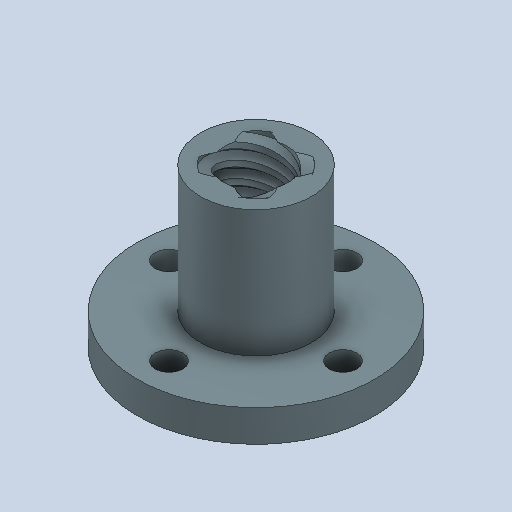
# Autodesk Inventor part: Nut
Saved by Autodesk Inventor 2024 (Build 280153000, 153)
## iProperties
Created: 2022-08-25
Part Number: Nut
Material: Lead
Document SubType Name: Modeling
Designer: Andrew
Density: 11.34 g/cm^3
Appearance: Lead
Author: Andrew
Autodesk Inventor part; units mm, degrees
ref_plane "YZ Plane" through (0, 0, 0) normal (1, 0, 0) x (0, 1, 0)
ref_plane "XZ Plane" through (0, 0, 0) normal (0, 1, 0) x (-1, 0, 0)
ref_plane "XY Plane" through (0, 0, 0) normal (0, 0, 1) x (1, 0, 0)
sketch "Sketch1" plane through (0, 0, 0) normal (0, 1, 0) x (-1, 0, 0)
  circle A0 centre (0, 0) radius 15
  circle A1 centre (0, 0) radius 11 construction
  circle A2 centre (0, 0) radius 7
  circle A3 centre (0, 0) radius 4
  circle A4 centre (11, 0) radius 1.75
  circle A5 centre (0, -11) radius 1.75
  circle A6 centre (-11, 0) radius 1.75
  circle A7 centre (0, 11) radius 1.75
  dimension "d1" = 22
  dimension "d0" = 30
  dimension "d2" = 14
  dimension "d3" = 8
  dimension "d4" = 3.5
  dimension "d7" = 360
  constraints: 7 centre point, 6 coincident, 1 horizontal alignment, 13 other
  measures "d0" diameter of A0
  measures "d2" diameter of A2
  measures "d3" diameter of A3
  measures "d4" diameter of A4
extrude "Extrusion1" add sketch "Sketch1" along normal blind 20 contours A2
extrude "Extrusion2" add sketch "Sketch1" along normal blind 4 contours A0
sketch "Sketch2" plane through (0, 0, 0) normal (1, 0, 0) x (0, 1, 0)
  line L0 (20, -2.634) -> (22, -2.634) construction
  line L1 (22, -2.634) -> (22, -6.366) construction
  line L2 (22, -6.366) -> (20, -6.366) construction
  line L3 (20, -6.366) -> (20, -2.634) construction
  line L4 (20, -4.5) -> (22, -4.5) construction
  line L5 (20, -4) -> (22, -4) construction
  line L6 (20, -3.75) -> (22, -3.75) construction
  line L7 (20, -5) -> (22, -5) construction
  line L8 (20, -5.25) -> (22, -5.25) construction
  line L9 (20, -2.634) -> (21, -6.366) construction
  line L10 (22, -2.634) -> (21, -6.366) construction
  line L11 (20.366, -4) -> (21.634, -4)
  line L12 (21.299, -5.25) -> (20.701, -5.25)
  line L13 (21.634, -4) -> (21.299, -5.25)
  line L14 (20.366, -4) -> (20.701, -5.25)
  line L15 (0, 0) -> (20, 0)
  line L16 (20, -7) -> (20, 7) projected
  dimension "d13" = 2
  dimension "d14" = 3.7321
  dimension "d15" = 0.5
  dimension "d16" = 0.75
  dimension "d17" = 9
  constraints: 32 end point, 12 point on line, 5 midpoint, 4 symmetric about line, 3 collinear, 3 perpendicular, 2 parallel, 1 horizontal
  measures "d13" distance of L2.start L3.start
  measures "d14" distance of L1.start L2.start
  measures "d15" distance between parallel lines of L5 L4
  measures "d16" distance between parallel lines of L6 L4
  measures "d17" diameter of L4 L15
coil "Coil1" sketch "Sketch2" operation cut axis through (0, 0, 0) along (0, -1, 0) pitch 8 turns 2.75 hand right
pattern_circular "Circular Pattern1" count 4 over 360 about axis through (0, 0, 0) along (0, 1, 0) of "Coil1"
equation "\"d14\" = 1.86603 * d13"
equation "\"d15\" = 0.25 * d13"
body "Solid1"
